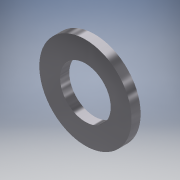
# Autodesk Inventor part: Part35
Saved by Autodesk Inventor 2017.3 (Build 213256000, 256)
## iProperties
Created: 2012-04-09
Part Number: Part35
Document SubType Name: Modeling
Designer: jhanson2
Density: 7.85 g/cm^3
Material: Steel
Appearance: Aluminum - Polished
Mass: 1.72046 g
Surface Area: 3.98834 cm^2
Volume: 0.219167 cm^3
Author: jhanson2
Autodesk Inventor part; units mm, degrees
ref_plane "YZ Plane" through (0, 0, 0) normal (1, 0, 0) x (0, 1, 0)
ref_plane "XZ Plane" through (0, 0, 0) normal (0, 1, 0) x (-1, 0, 0)
ref_plane "XY Plane" through (0, 0, 0) normal (0, 0, 1) x (1, 0, 0)
sketch "Sketch1" plane through (0, 0, 0) normal (0, 0, 1) x (1, 0, 0)
  circle A0 centre (0, 0) radius 4.3656
  circle A1 centre (0, 0) radius 7.9375
  dimension "d0" = 15.875
  dimension "d1" = 8.7312
  constraints: 2 centre point, 2 coincident
  measures "d0" diameter of A1
  measures "d1" diameter of A0
extrude "Extrusion1" add sketch "Sketch1" along normal blind 1.5875
body "Solid1"
